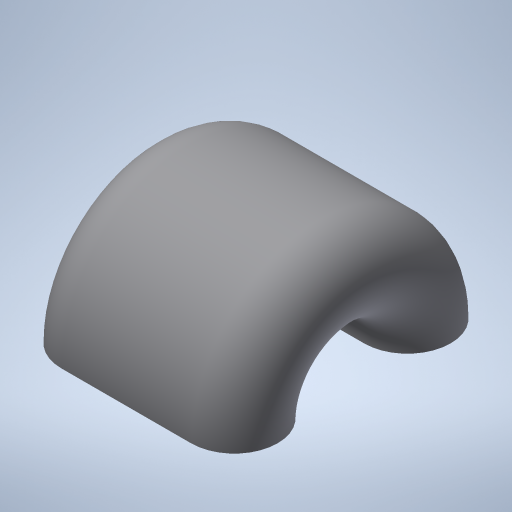
# Autodesk Inventor part: seguro
Saved by Autodesk Inventor 2023 (Build 270158000, 158)
## iProperties
Created: 2022-10-18
Part Number: seguro
Material: Generic
Document SubType Name: Modeling
Designer: Xiaba
Density: 1 g/cm^3
Appearance: Default
Author: Xiaba
Autodesk Inventor part; units mm, degrees
ref_plane "YZ Plane" through (0, 0, 0) normal (1, 0, 0) x (0, 1, 0)
ref_plane "XZ Plane" through (0, 0, 0) normal (0, 1, 0) x (-1, 0, 0)
ref_plane "XY Plane" through (0, 0, 0) normal (0, 0, 1) x (1, 0, 0)
sketch "Sketch1" plane through (0, 0, 0) normal (0, 1, 0) x (-1, 0, 0)
  line L0 (1.5, -1.6689) -> (-1.5, -1.6689)
  line L1 (-1.5, -3.6689) -> (1.5, -3.6689)
  arc A0 (2.5, -2.6689) -> (1.5, -1.6689) centre (1.5, -2.6689) ccw
  arc A1 (1.5, -3.6689) -> (2.5, -2.6689) centre (1.5, -2.6689) ccw
  arc A2 (-2.5, -2.6689) -> (-1.5, -3.6689) centre (-1.5, -2.6689) ccw
  arc A3 (-1.5, -1.6689) -> (-2.5, -2.6689) centre (-1.5, -2.6689) ccw
  line L2 (1.5, -2.6689) -> (-1.5, -2.6689) construction
  point P0 (2.5, -1.6689)
  point P1 (-2.5, -3.6689)
  point P2 (2.5, -3.6689)
  point P3 (-2.5, -2.6689)
  dimension "d1" = 5
  dimension "d2" = 2
  dimension "d3" = 1
  dimension "d4" = 1
  constraints: 8 point on circle, 6 end point, 4 centre point, 4 tangent, 3 point on line, 2 equal radius, 2 horizontal, 1 parallel, 13 other
  measures "d1" distance of point (-2.5, -3.669) point (2.5, -3.669)
  measures "d2" distance of point (2.5, -3.669) point (2.5, -1.669)
  measures "d3" radius of A0
  measures "d4" radius of A1
sketch "Sketch2" plane through (0, 0, 0) normal (1, 0, 0) x (0, 1, 0)
  line L0 (0, -2.6689) -> (0, 1.3311) construction
  arc A0 (0, -2.6689) -> (0, 1.3311) centre (0, -0.6689) ccw
  point P0 (0, 0)
  dimension "d5" = 4
  constraints: 2 end point, 2 point on circle, 1 centre point, 1 coincident, 1 midpoint, 1 vertical
  measures "d5" distance of L0.start L0.end
sweep "Sweep1" add profiles "Sketch1" path "Sketch2"
body "Solid1"
